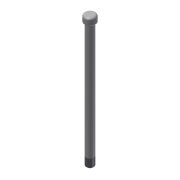
# Autodesk Inventor part: HANDLE
Saved by Autodesk Inventor 2014 (Build 180170000, 170)
## iProperties
Created: 2014-12-22
Part Number: HANDLE
Material: Steel, Mild
Document SubType Name: Modeling
Designer: Ebrahim
Density: 7.86 g/cm^3
Appearance: Steel
Mass: 386.553 g
Surface Area: 132.238 cm^2
Volume: 49.1797 cm^3
Author: Ebrahim
Autodesk Inventor part; units mm, degrees
ref_plane "YZ Plane" through (0, 0, 0) normal (1, 0, 0) x (0, 1, 0)
ref_plane "XZ Plane" through (0, 0, 0) normal (0, 1, 0) x (-1, 0, 0)
ref_plane "XY Plane" through (0, 0, 0) normal (0, 0, 1) x (1, 0, 0)
sketch "Sketch1" plane through (0, 0, 0) normal (0, 0, 1) x (1, 0, 0)
  circle A0 centre (0, 0) radius 7.5
  dimension "d0" = 15
  constraints: 1 centre point, 1 coincident
  measures "d0" diameter of A0
extrude "Extrusion1" add sketch "Sketch1" along normal mid plane 250
sketch "Sketch2" plane through (0, 0, 125) normal (0, 0, 1) x (1, 0, 0)
  circle A0 centre (0, 0) radius 7.5 projected
  circle A1 centre (0, 0) radius 11
  dimension "d3" = 22
  constraints: 1 centre point, 1 coincident
  measures "d3" diameter of A1
extrude "Extrusion2" add sketch "Sketch2" along normal blind 14 contours A0 | A1
fillet "Fillet1" radius 2 2 edges at (-11, 0, 125) (-7.5, 0, 125)
fillet "Fillet2" radius 4 1 edges at (-11, 0, 139)
chamfer "Chamfer1" distance 2 angle 45 1 edges at (-7.5, 0, -125)
thread "Thread1" size "M15x1" class "6g" standard "ISO Metric profile" length 16
body "Solid1"
